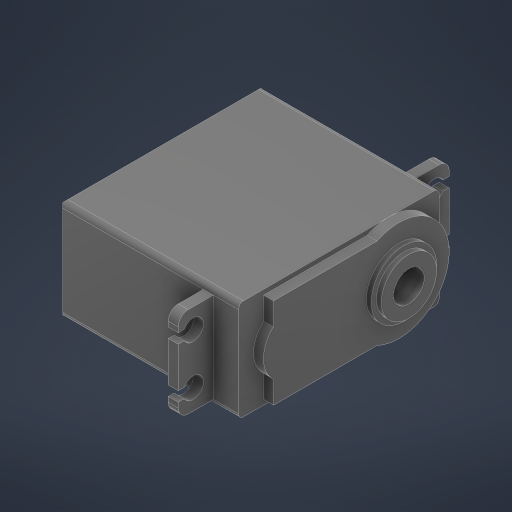
# Autodesk Inventor part: Servo
Saved by Autodesk Inventor 2023.2 (Build 272271000, 271)
## iProperties
Created: 2023-04-06
Part Number: Servo
Material: ABS-Kunststoff
Document SubType Name: Modeling
Designer: tadeus
Density: 1.06 g/cm^3
Appearance: Glatt - Weiß
Author: tadeus
Autodesk Inventor part; units mm, degrees
ref_plane "YZ Plane" through (0, 0, 0) normal (1, 0, 0) x (0, 1, 0)
ref_plane "XZ Plane" through (0, 0, 0) normal (0, 1, 0) x (-1, 0, 0)
ref_plane "XY Plane" through (0, 0, 0) normal (0, 0, 1) x (1, 0, 0)
sketch "Skizze1" plane through (0, 0, 0) normal (0, 1, 0) x (-1, 0, 0)
  line L0 (18.5, -20) -> (-18.5, -20)
  line L1 (-18.5, -20) -> (-18.5, 20)
  line L2 (-18.5, 20) -> (18.5, 20)
  line L3 (18.5, 20) -> (18.5, -20)
  line L4 (18.5, -20) -> (-18.5, 20) construction
  line L5 (-18.5, -20) -> (18.5, 20) construction
  point P0 (0, 0)
  dimension "d0" = 37
  dimension "d1" = 40
  constraints: 12 end point, 2 midpoint, 2 parallel, 1 horizontal, 1 perpendicular
  measures "d0" distance of L1.end L2.end
  measures "d1" distance of L0.end L1.end
extrude "Extrusion1" add sketch "Skizze1" along normal blind 20
sketch "Skizze2" plane through (0, 0, 0) normal (0, 0, 1) x (1, 0, 0)
  line L0 (-14.5, 13.5) -> (-10.5, 13.5)
  line L1 (-10.5, 13.5) -> (-10.5, 6.5)
  line L2 (-10.5, 6.5) -> (-14.5, 6.5)
  line L3 (-14.5, 6.5) -> (-14.5, 13.5)
  line L4 (-14.5, 13.5) -> (-10.5, 6.5) construction
  line L5 (-10.5, 13.5) -> (-14.5, 6.5) construction
  line L6 (-18.5, 20) -> (18.5, 20) projected
  line L7 (-18.5, 0) -> (-18.5, 20) projected
  line L8 (11.5, 19) -> (13.5, 19)
  line L9 (13.5, 19) -> (13.5, 1)
  line L10 (13.5, 1) -> (11.5, 1)
  line L11 (11.5, 1) -> (11.5, 19)
  line L12 (11.5, 19) -> (13.5, 1) construction
  line L13 (13.5, 19) -> (11.5, 1) construction
  line L14 (18.5, 0) -> (18.5, 20) projected
  point P0 (0, 0)
  point P1 (-12.5, 10)
  point P2 (12.5, 10)
  point P3 (18.5, 10)
  dimension "d4" = 4
  dimension "d5" = 7
  dimension "d6" = 10
  dimension "d7" = 6
  dimension "d10" = 2
  dimension "d11" = 18
  dimension "d12" = 6
  constraints: 24 end point, 5 midpoint, 4 parallel, 2 horizontal, 2 perpendicular
  measures "d4" distance of L1.end L2.end
  measures "d5" distance of L0.end L1.end
  measures "d6" distance from line of L6 point (-12.5, 10)
  measures "d7" distance from line of L7 point (-12.5, 10)
  measures "d10" distance of L9.end L10.end
  measures "d11" distance of L8.end L9.end
  measures "d12" distance of point (18.5, 10) point (12.5, 10)
extrude "Extrusion2" add sketch "Skizze2" against normal blind 5 from surface at -20 contours L0 L1 L2 L3
extrude "Extrusion3" add sketch "Skizze2" along normal mid plane 54 contours L8 L9 L10 L11
sketch "Skizze3" plane through (0, 0, 0) normal (1, 0, 0) x (0, 1, 0)
  arc A0 (15, 26.05) -> (14, 25.7896) centre (15, 24) ccw construction
  arc A1 (4, 25.7896) -> (6, 25.7896) centre (5, 24) ccw
  line L0 (1, 27) -> (19, 27) construction
  line L1 (15, 24) -> (5, 24) construction
  line L2 (19, 20) -> (19, 27) projected
  line L3 (-8.9518, 0) -> (31.8081, 0) construction
  line L4 (15, 24) -> (15, 27) construction
  line L5 (16, 25.1) -> (14, 25.1) construction
  line L6 (14, 25.1) -> (14, 25.7896)
  line L7 (14, 27) -> (16, 27)
  line L8 (16, 27) -> (16, 25.7896)
  line L9 (16, 25.1) -> (14, 27) construction
  line L10 (14, 25.1) -> (16, 27) construction
  line L11 (5, 24) -> (5, 27) construction
  line L12 (6, 25.1) -> (4, 25.1) construction
  line L13 (4, 25.1) -> (4, 25.7896) construction
  line L14 (4, 27) -> (6, 27)
  line L15 (6, 27) -> (6, 25.7896)
  line L16 (6, 25.1) -> (4, 27) construction
  line L17 (4, 25.1) -> (6, 27) construction
  line L18 (16, 25.7896) -> (16, 25.1) construction
  line L19 (14, 25.7896) -> (14, 27)
  arc A2 (16, 25.7896) -> (15, 26.05) centre (15, 24) ccw construction
  arc A3 (14, 25.7896) -> (16, 25.7896) centre (15, 24) ccw
  line L20 (6, 25.7896) -> (6, 25.1) construction
  line L21 (4, 25.7896) -> (4, 27)
  arc A4 (5, 26.05) -> (4, 25.7896) centre (5, 24) ccw construction
  arc A5 (6, 25.7896) -> (5, 26.05) centre (5, 24) ccw construction
  arc A6 (6, -25.7896) -> (4, -25.7896) centre (5, -24) ccw
  line L22 (14, -27) -> (16, -27)
  line L23 (16, -27) -> (16, -25.7896)
  line L24 (4, -27) -> (6, -27)
  line L25 (6, -27) -> (6, -25.7896)
  line L26 (14, -25.7896) -> (14, -27)
  arc A7 (16, -25.7896) -> (14, -25.7896) centre (15, -24) ccw
  line L27 (4, -25.7896) -> (4, -27)
  arc A8 (1, -5.6411) -> (19, -5.6411) centre (10, -10) ccw
  line L28 (20, 20) -> (20, -20) projected
  line L29 (0, -20) -> (20, -20) projected
  line L30 (19, -15) -> (1, -15) construction
  line L31 (1, -15) -> (1, -5.6411) construction
  line L32 (1, 15) -> (5.5, 15)
  line L33 (19, 15) -> (19, -5.6411)
  line L34 (19, -15) -> (1, 15) construction
  line L35 (1, -15) -> (19, 15) construction
  line L36 (0, 20) -> (20, 20) projected
  line L37 (19, -5.6411) -> (19, -15) construction
  line L38 (1, -5.6411) -> (1, 15)
  arc A9 (10, 0) -> (1, -5.6411) centre (10, -10) ccw construction
  arc A10 (19, -5.6411) -> (10, 0) centre (10, -10) ccw construction
  arc A11 (14.5, 15) -> (5.5, 15) centre (10, 10.9375) ccw
  line L39 (5.5, 15) -> (14.5, 15) construction
  line L40 (14.5, 15) -> (19, 15)
  point P0 (0, 0)
  point P1 (10, 15)
  point P2 (10, 17)
  dimension "d15" = 4.1
  dimension "d16" = 4.1
  dimension "d17" = 10
  dimension "d21" = 24
  dimension "d22" = 4
  dimension "d23" = 2
  dimension "d24" = 2
  dimension "d27" = 20
  dimension "d28" = 10
  dimension "d29" = 10
  dimension "d30" = 18
  dimension "d31" = 5
  dimension "d32" = 9
  dimension "d35" = 9
  dimension "d36" = 4.5
  dimension "d38" = 2
  constraints: 72 end point, 25 point on circle, 17 parallel, 12 centre point, 10 midpoint, 10 symmetric about line, 9 point on line, 8 perpendicular, 6 horizontal, 2 other
  measures "d15" diameter of A0
  measures "d16" diameter of A1
  measures "d17" distance of L1.end L1.start
  measures "d21" vertical distance of L1.end point (0, 0)
  measures "d22" distance from line of L2 L1.start
  measures "d23" distance of L7.start L7.end
  measures "d24" distance of L14.start L14.end
  measures "d27" diameter of A8
  measures "d28" distance from line of L28 A8.centre
  measures "d29" distance from line of L29 A8.centre
  measures "d30" distance of L32.start L33.start
  measures "d31" distance between parallel lines of L36 L32
  measures "d32" distance of L33.start point (10, 15)
  measures "d35" distance of L32.end L39.end
  measures "d36" distance of point (10, 15) L39.end
  measures "d38" distance from line of L32 point (10, 17)
extrude "Extrusion4" cut sketch "Skizze3" along normal through all contours L21 L14 L15 A1 | L7 L8 A3 L19 | L25 L24 L27 A6 | L26 A7 L23 L22
extrude "Extrusion5" add sketch "Skizze3" along normal blind 2 from surface at 18.5 contours L38 L32 A11 L40 L33 A8
sketch "Skizze4" plane through (20.5, 10, -10) normal (1, 0, 0) x (0, 0, -1)
  circle A0 centre (0, 0) radius 6.5
  circle A1 centre (0, 0) radius 5.5
  arc A2 (-4.3589, -9) -> (-4.3589, 9) centre (0, 0) ccw construction
  line L0 (0, 10) -> (10, 10) construction
  line L1 (0, 2.75) -> (0, 3) construction
  line L2 (-0.3447, 2.7283) -> (-0.376, 2.9763) construction
  line L3 (-0.6839, 2.6636) -> (-0.7461, 2.9057) construction
  line L4 (-1.0123, 2.5569) -> (-1.1044, 2.7893) construction
  line L5 (-1.3248, 2.4098) -> (-1.4453, 2.6289) construction
  line L6 (-1.6164, 2.2248) -> (-1.7634, 2.4271) construction
  line L7 (-1.8825, 2.0047) -> (-2.0536, 2.1869) construction
  line L8 (-2.1189, 1.7529) -> (-2.3115, 1.9123) construction
  line L9 (-2.3219, 1.4735) -> (-2.533, 1.6075) construction
  line L10 (-2.4883, 1.1709) -> (-2.7145, 1.2773) construction
  line L11 (-2.6154, 0.8498) -> (-2.8532, 0.9271) construction
  line L12 (-2.7013, 0.5153) -> (-2.9469, 0.5621) construction
  line L13 (-2.7446, 0.1727) -> (-2.9941, 0.1884) construction
  line L14 (-2.7446, -0.1727) -> (-2.9941, -0.1884) construction
  line L15 (-2.7013, -0.5153) -> (-2.9469, -0.5621) construction
  line L16 (-2.6154, -0.8498) -> (-2.8532, -0.9271) construction
  line L17 (-2.4883, -1.1709) -> (-2.7145, -1.2773) construction
  line L18 (-2.3219, -1.4735) -> (-2.533, -1.6075) construction
  line L19 (-2.1189, -1.7529) -> (-2.3115, -1.9123) construction
  line L20 (-1.8825, -2.0047) -> (-2.0536, -2.1869) construction
  line L21 (-1.6164, -2.2248) -> (-1.7634, -2.4271) construction
  line L22 (-1.3248, -2.4098) -> (-1.4453, -2.6289) construction
  line L23 (-1.0123, -2.5569) -> (-1.1044, -2.7893) construction
  line L24 (-0.6839, -2.6636) -> (-0.7461, -2.9057) construction
  line L25 (-0.3447, -2.7283) -> (-0.376, -2.9763) construction
  line L26 (0, -2.75) -> (0, -3) construction
  line L27 (0.3447, -2.7283) -> (0.376, -2.9763) construction
  line L28 (0.6839, -2.6636) -> (0.7461, -2.9057) construction
  line L29 (1.0123, -2.5569) -> (1.1044, -2.7893) construction
  line L30 (1.3248, -2.4098) -> (1.4453, -2.6289) construction
  line L31 (1.6164, -2.2248) -> (1.7634, -2.4271) construction
  line L32 (1.8825, -2.0047) -> (2.0536, -2.1869) construction
  line L33 (2.1189, -1.7529) -> (2.3115, -1.9123) construction
  line L34 (2.3219, -1.4735) -> (2.533, -1.6075) construction
  line L35 (2.4883, -1.1709) -> (2.7145, -1.2773) construction
  line L36 (2.6154, -0.8498) -> (2.8532, -0.9271) construction
  line L37 (2.7013, -0.5153) -> (2.9469, -0.5621) construction
  line L38 (2.7446, -0.1727) -> (2.9941, -0.1884) construction
  line L39 (2.7446, 0.1727) -> (2.9941, 0.1884) construction
  line L40 (2.7013, 0.5153) -> (2.9469, 0.5621) construction
  line L41 (2.6154, 0.8498) -> (2.8532, 0.9271) construction
  line L42 (2.4883, 1.1709) -> (2.7145, 1.2773) construction
  line L43 (2.3219, 1.4735) -> (2.533, 1.6075) construction
  line L44 (2.1189, 1.7529) -> (2.3115, 1.9123) construction
  line L45 (1.8825, 2.0047) -> (2.0536, 2.1869) construction
  line L46 (1.6164, 2.2248) -> (1.7634, 2.4271) construction
  line L47 (1.3248, 2.4098) -> (1.4453, 2.6289) construction
  line L48 (1.0123, 2.5569) -> (1.1044, 2.7893) construction
  line L49 (0.6839, 2.6636) -> (0.7461, 2.9057) construction
  line L50 (0.3447, 2.7283) -> (0.376, 2.9763) construction
  spline S0 degree 4 poles (0, 3) (0.1244, 3) (0.1756, 2.8504) (0.2331, 2.7424) (0.3447, 2.7283) knots 0 0 0 0 0 1 1 1 1 1
  line L51 (0.3012, 2.7338) -> (0.3881, 2.7228) construction
  arc A3 (0.3111, 2.7361) -> (0.3791, 2.7275) centre (0.3658, 2.8957) ccw construction
  line L52 (-0.0449, 3) -> (0.0449, 3) construction
  arc A4 (0.0348, 2.9956) -> (-0.0348, 2.9956) centre (0, 2.862) ccw construction
  spline S1 degree 4 poles (0, 3) (-0.1244, 3) (-0.1756, 2.8504) (-0.2331, 2.7424) (-0.3447, 2.7283) knots 0 0 0 0 0 1 1 1 1 1
  line L53 (-0.3012, 2.7338) -> (-0.3881, 2.7228) construction
  arc A5 (-0.3791, 2.7275) -> (-0.3111, 2.7361) centre (-0.3658, 2.8957) ccw construction
  line L54 (0.0449, 3) -> (-0.0449, 3) construction
  arc A6 (0.0348, 2.9956) -> (-0.0348, 2.9956) centre (0, 2.862) ccw construction
  spline S2 degree 4 poles (-0.7461, 2.9057) (-0.6256, 2.9367) (-0.5388, 2.8045) (-0.4562, 2.7142) (-0.3447, 2.7283) knots 0 0 0 0 0 1 1 1 1 1
  line L55 (-0.3881, 2.7228) -> (-0.3012, 2.7338) construction
  line L56 (-0.7895, 2.8946) -> (-0.7026, 2.9169) construction
  arc A7 (-0.3791, 2.7275) -> (-0.3111, 2.7361) centre (-0.3658, 2.8957) ccw construction
  arc A8 (-0.7113, 2.9101) -> (-0.7786, 2.8928) centre (-0.7118, 2.7721) ccw construction
  spline S3 degree 4 poles (-0.7461, 2.9057) (-0.8666, 2.8748) (-0.879, 2.7172) (-0.9078, 2.5983) (-1.0123, 2.5569) knots 0 0 0 0 0 1 1 1 1 1
  line L57 (-0.9716, 2.573) -> (-1.0531, 2.5408) construction
  line L58 (-0.7026, 2.9169) -> (-0.7895, 2.8946) construction
  arc A9 (-1.0455, 2.5475) -> (-0.9817, 2.5728) centre (-1.0745, 2.7138) ccw construction
  arc A10 (-0.7113, 2.9101) -> (-0.7786, 2.8928) centre (-0.7118, 2.7721) ccw construction
  spline S4 degree 4 poles (-1.4453, 2.6289) (-1.3362, 2.6889) (-1.2193, 2.5824) (-1.1169, 2.5155) (-1.0123, 2.5569) knots 0 0 0 0 0 1 1 1 1 1
  line L59 (-1.0531, 2.5408) -> (-0.9716, 2.573) construction
  line L60 (-1.4846, 2.6073) -> (-1.4059, 2.6505) construction
  arc A11 (-1.0455, 2.5475) -> (-0.9817, 2.5728) centre (-1.0745, 2.7138) ccw construction
  arc A12 (-1.4127, 2.6418) -> (-1.4736, 2.6083) centre (-1.3788, 2.508) ccw construction
  spline S5 degree 4 poles (-1.4453, 2.6289) (-1.5543, 2.569) (-1.5271, 2.4132) (-1.5254, 2.2909) (-1.6164, 2.2248) knots 0 0 0 0 0 1 1 1 1 1
  line L61 (-1.581, 2.2505) -> (-1.6518, 2.1991) construction
  line L62 (-1.4059, 2.6505) -> (-1.4846, 2.6073) construction
  arc A13 (-1.6462, 2.2075) -> (-1.5907, 2.2478) centre (-1.7156, 2.3613) ccw construction
  arc A14 (-1.4127, 2.6418) -> (-1.4736, 2.6083) centre (-1.3788, 2.508) ccw construction
  spline S6 degree 4 poles (-2.0536, 2.1869) (-1.9629, 2.2721) (-1.8232, 2.1981) (-1.7074, 2.1587) (-1.6164, 2.2248) knots 0 0 0 0 0 1 1 1 1 1
  line L63 (-1.6518, 2.1991) -> (-1.581, 2.2505) construction
  line L64 (-2.0864, 2.1562) -> (-2.0209, 2.2176) construction
  arc A15 (-1.6462, 2.2075) -> (-1.5907, 2.2478) centre (-1.7156, 2.3613) ccw construction
  arc A16 (-2.0253, 2.2075) -> (-2.0759, 2.1599) centre (-1.9592, 2.0863) ccw construction
  spline S7 degree 4 poles (-2.0536, 2.1869) (-2.1443, 2.1017) (-2.0792, 1.9576) (-2.0472, 1.8396) (-2.1189, 1.7529) knots 0 0 0 0 0 1 1 1 1 1
  line L65 (-2.091, 1.7867) -> (-2.1468, 1.7192) construction
  line L66 (-2.0209, 2.2176) -> (-2.0864, 2.1562) construction
  arc A17 (-2.1435, 1.7287) -> (-2.0998, 1.7816) centre (-2.2489, 1.8605) ccw construction
  arc A18 (-2.0253, 2.2075) -> (-2.0759, 2.1599) centre (-1.9592, 2.0863) ccw construction
  spline S8 degree 4 poles (-2.533, 1.6075) (-2.4663, 1.7125) (-2.3126, 1.6756) (-2.1906, 1.6663) (-2.1189, 1.7529) knots 0 0 0 0 0 1 1 1 1 1
  line L67 (-2.1468, 1.7192) -> (-2.091, 1.7867) construction
  line L68 (-2.557, 1.5696) -> (-2.5089, 1.6454) construction
  arc A19 (-2.1435, 1.7287) -> (-2.0998, 1.7816) centre (-2.2489, 1.8605) ccw construction
  arc A20 (-2.5106, 1.6344) -> (-2.5478, 1.5758) centre (-2.4165, 1.5335) ccw construction
  spline S9 degree 4 poles (-2.533, 1.6075) (-2.5997, 1.5024) (-2.5008, 1.3791) (-2.4404, 1.2727) (-2.4883, 1.1709) knots 0 0 0 0 0 1 1 1 1 1
  line L69 (-2.4696, 1.2105) -> (-2.5069, 1.1313) construction
  line L70 (-2.5089, 1.6454) -> (-2.557, 1.5696) construction
  arc A21 (-2.5061, 1.1414) -> (-2.4769, 1.2034) centre (-2.641, 1.2427) ccw construction
  arc A22 (-2.5106, 1.6344) -> (-2.5478, 1.5758) centre (-2.4165, 1.5335) ccw construction
  spline S10 degree 4 poles (-2.8532, 0.9271) (-2.8147, 1.0454) (-2.6566, 1.0478) (-2.5362, 1.0691) (-2.4883, 1.1709) knots 0 0 0 0 0 1 1 1 1 1
  line L71 (-2.5069, 1.1313) -> (-2.4696, 1.2105) construction
  line L72 (-2.867, 0.8844) -> (-2.8393, 0.9697) construction
  arc A23 (-2.5061, 1.1414) -> (-2.4769, 1.2034) centre (-2.641, 1.2427) ccw construction
  arc A24 (-2.8382, 0.9587) -> (-2.8597, 0.8926) centre (-2.7219, 0.8844) ccw construction
  spline S11 degree 4 poles (-2.8532, 0.9271) (-2.8916, 0.8087) (-2.7652, 0.7138) (-2.6802, 0.6258) (-2.7013, 0.5153) knots 0 0 0 0 0 1 1 1 1 1
  line L73 (-2.6931, 0.5583) -> (-2.7095, 0.4723) construction
  line L74 (-2.8393, 0.9697) -> (-2.867, 0.8844) construction
  arc A25 (-2.7112, 0.4823) -> (-2.6983, 0.5497) centre (-2.867, 0.5469) ccw construction
  arc A26 (-2.8382, 0.9587) -> (-2.8597, 0.8926) centre (-2.7219, 0.8844) ccw construction
  spline S12 degree 4 poles (-2.9941, 0.1884) (-2.9863, 0.3125) (-2.8338, 0.3542) (-2.7224, 0.4048) (-2.7013, 0.5153) knots 0 0 0 0 0 1 1 1 1 1
  line L75 (-2.7095, 0.4723) -> (-2.6931, 0.5583) construction
  line L76 (-2.9969, 0.1436) -> (-2.9913, 0.2332) construction
  arc A27 (-2.7112, 0.4823) -> (-2.6983, 0.5497) centre (-2.867, 0.5469) ccw construction
  arc A28 (-2.9875, 0.2228) -> (-2.9918, 0.1534) centre (-2.8564, 0.1797) ccw construction
  spline S13 degree 4 poles (-2.9941, 0.1884) (-3.0019, 0.0642) (-2.8558, 0.0037) (-2.7516, -0.0604) (-2.7446, -0.1727) knots 0 0 0 0 0 1 1 1 1 1
  line L77 (-2.7473, -0.129) -> (-2.7418, -0.2164) construction
  line L78 (-2.9913, 0.2332) -> (-2.9969, 0.1436) construction
  arc A29 (-2.7459, -0.2071) -> (-2.7502, -0.1387) centre (-2.913, -0.1833) ccw construction
  arc A30 (-2.9875, 0.2228) -> (-2.9918, 0.1534) centre (-2.8564, 0.1797) ccw construction
  spline S14 degree 4 poles (-2.9469, -0.5621) (-2.9702, -0.4399) (-2.8328, -0.3616) (-2.7375, -0.2849) (-2.7446, -0.1727) knots 0 0 0 0 0 1 1 1 1 1
  line L79 (-2.7418, -0.2164) -> (-2.7473, -0.129) construction
  line L80 (-2.9385, -0.6062) -> (-2.9553, -0.518) construction
  arc A31 (-2.7459, -0.2071) -> (-2.7502, -0.1387) centre (-2.913, -0.1833) ccw construction
  arc A32 (-2.949, -0.5272) -> (-2.936, -0.5954) centre (-2.8113, -0.5363) ccw construction
  spline S15 degree 4 poles (-2.9469, -0.5621) (-2.9235, -0.6844) (-2.767, -0.7066) (-2.6502, -0.7428) (-2.6154, -0.8498) knots 0 0 0 0 0 1 1 1 1 1
  line L81 (-2.6289, -0.8081) -> (-2.6019, -0.8914) construction
  line L82 (-2.9553, -0.518) -> (-2.9385, -0.6062) construction
  arc A33 (-2.6082, -0.8835) -> (-2.6294, -0.8183) centre (-2.7759, -0.9019) ccw construction
  arc A34 (-2.949, -0.5272) -> (-2.936, -0.5954) centre (-2.8113, -0.5363) ccw construction
  spline S16 degree 4 poles (-2.7145, -1.2773) (-2.7675, -1.1648) (-2.6539, -1.0548) (-2.5807, -0.9568) (-2.6154, -0.8498) knots 0 0 0 0 0 1 1 1 1 1
  line L83 (-2.6019, -0.8914) -> (-2.6289, -0.8081) construction
  line L84 (-2.6954, -1.318) -> (-2.7336, -1.2367) construction
  arc A35 (-2.6082, -0.8835) -> (-2.6294, -0.8183) centre (-2.7759, -0.9019) ccw construction
  arc A36 (-2.7253, -1.244) -> (-2.6957, -1.3069) centre (-2.5896, -1.2186) ccw construction
  spline S17 degree 4 poles (-2.7145, -1.2773) (-2.6615, -1.3899) (-2.5044, -1.3725) (-2.3822, -1.3786) (-2.3219, -1.4735) knots 0 0 0 0 0 1 1 1 1 1
  line L85 (-2.3454, -1.4365) -> (-2.2984, -1.5105) construction
  line L86 (-2.7336, -1.2367) -> (-2.6954, -1.318) construction
  arc A37 (-2.3065, -1.5044) -> (-2.3433, -1.4464) centre (-2.4644, -1.5639) ccw construction
  arc A38 (-2.7253, -1.244) -> (-2.6957, -1.3069) centre (-2.5896, -1.2186) ccw construction
  spline S18 degree 4 poles (-2.3115, -1.9123) (-2.3908, -1.8164) (-2.3082, -1.6816) (-2.2616, -1.5685) (-2.3219, -1.4735) knots 0 0 0 0 0 1 1 1 1 1
  line L87 (-2.2984, -1.5105) -> (-2.3454, -1.4365) construction
  line L88 (-2.2829, -1.9469) -> (-2.3402, -1.8777) construction
  arc A39 (-2.3065, -1.5044) -> (-2.3433, -1.4464) centre (-2.4644, -1.5639) ccw construction
  arc A40 (-2.3303, -1.8827) -> (-2.286, -1.9362) centre (-2.2052, -1.8243) ccw construction
  spline S19 degree 4 poles (-2.3115, -1.9123) (-2.2322, -2.0081) (-2.0843, -1.9522) (-1.9645, -1.9277) (-1.8825, -2.0047) knots 0 0 0 0 0 1 1 1 1 1
  line L89 (-1.9144, -1.9747) -> (-1.8506, -2.0346) construction
  line L90 (-2.3402, -1.8777) -> (-2.2829, -1.9469) construction
  arc A41 (-1.8599, -2.0307) -> (-1.9099, -1.9838) centre (-1.998, -2.1277) ccw construction
  arc A42 (-2.3303, -1.8827) -> (-2.286, -1.9362) centre (-2.2052, -1.8243) ccw construction
  spline S20 degree 4 poles (-1.7634, -2.4271) (-1.864, -2.3539) (-1.8175, -2.2028) (-1.8005, -2.0817) (-1.8825, -2.0047) knots 0 0 0 0 0 1 1 1 1 1
  line L91 (-1.8506, -2.0346) -> (-1.9144, -1.9747) construction
  line L92 (-1.727, -2.4534) -> (-1.7997, -2.4007) construction
  arc A43 (-1.8599, -2.0307) -> (-1.9099, -1.9838) centre (-1.998, -2.1277) ccw construction
  arc A44 (-1.7889, -2.403) -> (-1.7326, -2.4439) centre (-1.6823, -2.3154) ccw construction
  spline S21 degree 4 poles (-1.7634, -2.4271) (-1.6627, -2.5002) (-1.5334, -2.4092) (-1.4234, -2.3557) (-1.3248, -2.4098) knots 0 0 0 0 0 1 1 1 1 1
  line L93 (-1.3632, -2.3887) -> (-1.2864, -2.4309) construction
  line L94 (-1.7997, -2.4007) -> (-1.727, -2.4534) construction
  arc A45 (-1.2965, -2.4295) -> (-1.3566, -2.3964) centre (-1.4061, -2.5577) ccw construction
  arc A46 (-1.7889, -2.403) -> (-1.7326, -2.4439) centre (-1.6823, -2.3154) ccw construction
  spline S22 degree 4 poles (-1.1044, -2.7893) (-1.2201, -2.7435) (-1.2126, -2.5856) (-1.2263, -2.464) (-1.3248, -2.4098) knots 0 0 0 0 0 1 1 1 1 1
  line L95 (-1.2864, -2.4309) -> (-1.3632, -2.3887) construction
  line L96 (-1.0626, -2.8059) -> (-1.1461, -2.7728) construction
  arc A47 (-1.2965, -2.4295) -> (-1.3566, -2.3964) centre (-1.4061, -2.5577) ccw construction
  arc A48 (-1.135, -2.7724) -> (-1.0704, -2.798) centre (-1.0536, -2.661) ccw construction
  spline S23 degree 4 poles (-1.1044, -2.7893) (-0.9887, -2.8351) (-0.886, -2.7149) (-0.7928, -2.6356) (-0.6839, -2.6636) knots 0 0 0 0 0 1 1 1 1 1
  line L97 (-0.7263, -2.6527) -> (-0.6415, -2.6745) construction
  line L98 (-1.1461, -2.7728) -> (-1.0626, -2.8059) construction
  arc A49 (-0.6515, -2.6755) -> (-0.718, -2.6585) centre (-0.7259, -2.827) ccw construction
  arc A50 (-1.135, -2.7724) -> (-1.0704, -2.798) centre (-1.0536, -2.661) ccw construction
  spline S24 degree 4 poles (-0.376, -2.9763) (-0.4994, -2.9607) (-0.5315, -2.8059) (-0.575, -2.6916) (-0.6839, -2.6636) knots 0 0 0 0 0 1 1 1 1 1
  line L99 (-0.6415, -2.6745) -> (-0.7263, -2.6527) construction
  line L100 (-0.3315, -2.982) -> (-0.4205, -2.9707) construction
  arc A51 (-0.6515, -2.6755) -> (-0.718, -2.6585) centre (-0.7259, -2.827) ccw construction
  arc A52 (-0.4099, -2.9676) -> (-0.341, -2.9763) centre (-0.3587, -2.8395) ccw construction
  spline S25 degree 4 poles (-0.376, -2.9763) (-0.2526, -2.9919) (-0.183, -2.8499) (-0.1125, -2.75) (0, -2.75) knots 0 0 0 0 0 1 1 1 1 1
  line L101 (-0.0438, -2.75) -> (0.0438, -2.75) construction
  line L102 (-0.4205, -2.9707) -> (-0.3315, -2.982) construction
  arc A53 (0.0343, -2.7535) -> (-0.0343, -2.7535) centre (0, -2.9187) ccw construction
  arc A54 (-0.4099, -2.9676) -> (-0.341, -2.9763) centre (-0.3587, -2.8395) ccw construction
  spline S26 degree 4 poles (0.376, -2.9763) (0.2526, -2.9919) (0.183, -2.8499) (0.1125, -2.75) (0, -2.75) knots 0 0 0 0 0 1 1 1 1 1
  line L103 (0.0438, -2.75) -> (-0.0438, -2.75) construction
  line L104 (0.4205, -2.9707) -> (0.3315, -2.982) construction
  arc A55 (0.0343, -2.7535) -> (-0.0343, -2.7535) centre (0, -2.9187) ccw construction
  arc A56 (0.341, -2.9763) -> (0.4099, -2.9676) centre (0.3587, -2.8395) ccw construction
  spline S27 degree 4 poles (0.376, -2.9763) (0.4994, -2.9607) (0.5315, -2.8059) (0.575, -2.6916) (0.6839, -2.6636) knots 0 0 0 0 0 1 1 1 1 1
  line L105 (0.6415, -2.6745) -> (0.7263, -2.6527) construction
  line L106 (0.3315, -2.982) -> (0.4205, -2.9707) construction
  arc A57 (0.718, -2.6585) -> (0.6515, -2.6755) centre (0.7259, -2.827) ccw construction
  arc A58 (0.341, -2.9763) -> (0.4099, -2.9676) centre (0.3587, -2.8395) ccw construction
  spline S28 degree 4 poles (1.1044, -2.7893) (0.9887, -2.8351) (0.886, -2.7149) (0.7928, -2.6356) (0.6839, -2.6636) knots 0 0 0 0 0 1 1 1 1 1
  line L107 (0.7263, -2.6527) -> (0.6415, -2.6745) construction
  line L108 (1.1461, -2.7728) -> (1.0626, -2.8059) construction
  arc A59 (0.718, -2.6585) -> (0.6515, -2.6755) centre (0.7259, -2.827) ccw construction
  arc A60 (1.0704, -2.798) -> (1.135, -2.7724) centre (1.0536, -2.661) ccw construction
  spline S29 degree 4 poles (1.1044, -2.7893) (1.2201, -2.7435) (1.2126, -2.5856) (1.2263, -2.464) (1.3248, -2.4098) knots 0 0 0 0 0 1 1 1 1 1
  line L109 (1.2864, -2.4309) -> (1.3632, -2.3887) construction
  line L110 (1.0626, -2.8059) -> (1.1461, -2.7728) construction
  arc A61 (1.3566, -2.3964) -> (1.2965, -2.4295) centre (1.4061, -2.5577) ccw construction
  arc A62 (1.0704, -2.798) -> (1.135, -2.7724) centre (1.0536, -2.661) ccw construction
  spline S30 degree 4 poles (1.7634, -2.4271) (1.6627, -2.5002) (1.5334, -2.4092) (1.4234, -2.3557) (1.3248, -2.4098) knots 0 0 0 0 0 1 1 1 1 1
  line L111 (1.3632, -2.3887) -> (1.2864, -2.4309) construction
  line L112 (1.7997, -2.4007) -> (1.727, -2.4534) construction
  arc A63 (1.3566, -2.3964) -> (1.2965, -2.4295) centre (1.4061, -2.5577) ccw construction
  arc A64 (1.7326, -2.4439) -> (1.7889, -2.403) centre (1.6823, -2.3154) ccw construction
  spline S31 degree 4 poles (1.7634, -2.4271) (1.864, -2.3539) (1.8175, -2.2028) (1.8005, -2.0817) (1.8825, -2.0047) knots 0 0 0 0 0 1 1 1 1 1
  line L113 (1.8506, -2.0346) -> (1.9144, -1.9747) construction
  line L114 (1.727, -2.4534) -> (1.7997, -2.4007) construction
  arc A65 (1.9099, -1.9838) -> (1.8599, -2.0307) centre (1.998, -2.1277) ccw construction
  arc A66 (1.7326, -2.4439) -> (1.7889, -2.403) centre (1.6823, -2.3154) ccw construction
  spline S32 degree 4 poles (2.3115, -1.9123) (2.2322, -2.0081) (2.0843, -1.9522) (1.9645, -1.9277) (1.8825, -2.0047) knots 0 0 0 0 0 1 1 1 1 1
  line L115 (1.9144, -1.9747) -> (1.8506, -2.0346) construction
  line L116 (2.3402, -1.8777) -> (2.2829, -1.9469) construction
  arc A67 (1.9099, -1.9838) -> (1.8599, -2.0307) centre (1.998, -2.1277) ccw construction
  arc A68 (2.286, -1.9362) -> (2.3303, -1.8827) centre (2.2052, -1.8243) ccw construction
  spline S33 degree 4 poles (2.3115, -1.9123) (2.3908, -1.8164) (2.3082, -1.6816) (2.2616, -1.5685) (2.3219, -1.4735) knots 0 0 0 0 0 1 1 1 1 1
  line L117 (2.2984, -1.5105) -> (2.3454, -1.4365) construction
  line L118 (2.2829, -1.9469) -> (2.3402, -1.8777) construction
  arc A69 (2.3433, -1.4464) -> (2.3065, -1.5044) centre (2.4644, -1.5639) ccw construction
  arc A70 (2.286, -1.9362) -> (2.3303, -1.8827) centre (2.2052, -1.8243) ccw construction
  spline S34 degree 4 poles (2.7145, -1.2773) (2.6615, -1.3899) (2.5044, -1.3725) (2.3822, -1.3786) (2.3219, -1.4735) knots 0 0 0 0 0 1 1 1 1 1
  line L119 (2.3454, -1.4365) -> (2.2984, -1.5105) construction
  line L120 (2.7336, -1.2367) -> (2.6954, -1.318) construction
  arc A71 (2.3433, -1.4464) -> (2.3065, -1.5044) centre (2.4644, -1.5639) ccw construction
  arc A72 (2.6957, -1.3069) -> (2.7253, -1.244) centre (2.5896, -1.2186) ccw construction
  spline S35 degree 4 poles (2.7145, -1.2773) (2.7675, -1.1648) (2.6539, -1.0548) (2.5807, -0.9568) (2.6154, -0.8498) knots 0 0 0 0 0 1 1 1 1 1
  line L121 (2.6019, -0.8914) -> (2.6289, -0.8081) construction
  line L122 (2.6954, -1.318) -> (2.7336, -1.2367) construction
  arc A73 (2.6294, -0.8183) -> (2.6082, -0.8835) centre (2.7759, -0.9019) ccw construction
  arc A74 (2.6957, -1.3069) -> (2.7253, -1.244) centre (2.5896, -1.2186) ccw construction
  spline S36 degree 4 poles (2.9469, -0.5621) (2.9235, -0.6844) (2.767, -0.7066) (2.6502, -0.7428) (2.6154, -0.8498) knots 0 0 0 0 0 1 1 1 1 1
  line L123 (2.6289, -0.8081) -> (2.6019, -0.8914) construction
  line L124 (2.9553, -0.518) -> (2.9385, -0.6062) construction
  arc A75 (2.6294, -0.8183) -> (2.6082, -0.8835) centre (2.7759, -0.9019) ccw construction
  arc A76 (2.936, -0.5954) -> (2.949, -0.5272) centre (2.8113, -0.5363) ccw construction
  spline S37 degree 4 poles (2.9469, -0.5621) (2.9702, -0.4399) (2.8328, -0.3616) (2.7375, -0.2849) (2.7446, -0.1727) knots 0 0 0 0 0 1 1 1 1 1
  line L125 (2.7418, -0.2164) -> (2.7473, -0.129) construction
  line L126 (2.9385, -0.6062) -> (2.9553, -0.518) construction
  arc A77 (2.7502, -0.1387) -> (2.7459, -0.2071) centre (2.913, -0.1833) ccw construction
  arc A78 (2.936, -0.5954) -> (2.949, -0.5272) centre (2.8113, -0.5363) ccw construction
  spline S38 degree 4 poles (2.9941, 0.1884) (3.0019, 0.0642) (2.8558, 0.0037) (2.7516, -0.0604) (2.7446, -0.1727) knots 0 0 0 0 0 1 1 1 1 1
  line L127 (2.7473, -0.129) -> (2.7418, -0.2164) construction
  line L128 (2.9913, 0.2332) -> (2.9969, 0.1436) construction
  arc A79 (2.7502, -0.1387) -> (2.7459, -0.2071) centre (2.913, -0.1833) ccw construction
  arc A80 (2.9918, 0.1534) -> (2.9875, 0.2228) centre (2.8564, 0.1797) ccw construction
  spline S39 degree 4 poles (2.9941, 0.1884) (2.9863, 0.3125) (2.8338, 0.3542) (2.7224, 0.4048) (2.7013, 0.5153) knots 0 0 0 0 0 1 1 1 1 1
  line L129 (2.7095, 0.4723) -> (2.6931, 0.5583) construction
  line L130 (2.9969, 0.1436) -> (2.9913, 0.2332) construction
  arc A81 (2.6983, 0.5497) -> (2.7112, 0.4823) centre (2.867, 0.5469) ccw construction
  arc A82 (2.9918, 0.1534) -> (2.9875, 0.2228) centre (2.8564, 0.1797) ccw construction
  spline S40 degree 4 poles (2.8532, 0.9271) (2.8916, 0.8087) (2.7652, 0.7138) (2.6802, 0.6258) (2.7013, 0.5153) knots 0 0 0 0 0 1 1 1 1 1
  line L131 (2.6931, 0.5583) -> (2.7095, 0.4723) construction
  line L132 (2.8393, 0.9697) -> (2.867, 0.8844) construction
  arc A83 (2.6983, 0.5497) -> (2.7112, 0.4823) centre (2.867, 0.5469) ccw construction
  arc A84 (2.8597, 0.8926) -> (2.8382, 0.9587) centre (2.7219, 0.8844) ccw construction
  spline S41 degree 4 poles (2.8532, 0.9271) (2.8147, 1.0454) (2.6566, 1.0478) (2.5362, 1.0691) (2.4883, 1.1709) knots 0 0 0 0 0 1 1 1 1 1
  line L133 (2.5069, 1.1313) -> (2.4696, 1.2105) construction
  line L134 (2.867, 0.8844) -> (2.8393, 0.9697) construction
  arc A85 (2.4769, 1.2034) -> (2.5061, 1.1414) centre (2.641, 1.2427) ccw construction
  arc A86 (2.8597, 0.8926) -> (2.8382, 0.9587) centre (2.7219, 0.8844) ccw construction
  spline S42 degree 4 poles (2.533, 1.6075) (2.5997, 1.5024) (2.5008, 1.3791) (2.4404, 1.2727) (2.4883, 1.1709) knots 0 0 0 0 0 1 1 1 1 1
  line L135 (2.4696, 1.2105) -> (2.5069, 1.1313) construction
  line L136 (2.5089, 1.6454) -> (2.557, 1.5696) construction
  arc A87 (2.4769, 1.2034) -> (2.5061, 1.1414) centre (2.641, 1.2427) ccw construction
  arc A88 (2.5478, 1.5758) -> (2.5106, 1.6344) centre (2.4165, 1.5335) ccw construction
  spline S43 degree 4 poles (2.533, 1.6075) (2.4663, 1.7125) (2.3126, 1.6756) (2.1906, 1.6663) (2.1189, 1.7529) knots 0 0 0 0 0 1 1 1 1 1
  line L137 (2.1468, 1.7192) -> (2.091, 1.7867) construction
  line L138 (2.557, 1.5696) -> (2.5089, 1.6454) construction
  arc A89 (2.0998, 1.7816) -> (2.1435, 1.7287) centre (2.2489, 1.8605) ccw construction
  arc A90 (2.5478, 1.5758) -> (2.5106, 1.6344) centre (2.4165, 1.5335) ccw construction
  spline S44 degree 4 poles (2.0536, 2.1869) (2.1443, 2.1017) (2.0792, 1.9576) (2.0472, 1.8396) (2.1189, 1.7529) knots 0 0 0 0 0 1 1 1 1 1
  line L139 (2.091, 1.7867) -> (2.1468, 1.7192) construction
  line L140 (2.0209, 2.2176) -> (2.0864, 2.1562) construction
  arc A91 (2.0998, 1.7816) -> (2.1435, 1.7287) centre (2.2489, 1.8605) ccw construction
  arc A92 (2.0759, 2.1599) -> (2.0253, 2.2075) centre (1.9592, 2.0863) ccw construction
  spline S45 degree 4 poles (2.0536, 2.1869) (1.9629, 2.2721) (1.8232, 2.1981) (1.7074, 2.1587) (1.6164, 2.2248) knots 0 0 0 0 0 1 1 1 1 1
  line L141 (1.6518, 2.1991) -> (1.581, 2.2505) construction
  line L142 (2.0864, 2.1562) -> (2.0209, 2.2176) construction
  arc A93 (1.5907, 2.2478) -> (1.6462, 2.2075) centre (1.7156, 2.3613) ccw construction
  arc A94 (2.0759, 2.1599) -> (2.0253, 2.2075) centre (1.9592, 2.0863) ccw construction
  spline S46 degree 4 poles (1.4453, 2.6289) (1.5543, 2.569) (1.5271, 2.4132) (1.5254, 2.2909) (1.6164, 2.2248) knots 0 0 0 0 0 1 1 1 1 1
  line L143 (1.581, 2.2505) -> (1.6518, 2.1991) construction
  line L144 (1.4059, 2.6505) -> (1.4846, 2.6073) construction
  arc A95 (1.5907, 2.2478) -> (1.6462, 2.2075) centre (1.7156, 2.3613) ccw construction
  arc A96 (1.4736, 2.6083) -> (1.4127, 2.6418) centre (1.3788, 2.508) ccw construction
  spline S47 degree 4 poles (1.4453, 2.6289) (1.3362, 2.6889) (1.2193, 2.5824) (1.1169, 2.5155) (1.0123, 2.5569) knots 0 0 0 0 0 1 1 1 1 1
  line L145 (1.0531, 2.5408) -> (0.9716, 2.573) construction
  line L146 (1.4846, 2.6073) -> (1.4059, 2.6505) construction
  arc A97 (0.9817, 2.5728) -> (1.0455, 2.5475) centre (1.0745, 2.7138) ccw construction
  arc A98 (1.4736, 2.6083) -> (1.4127, 2.6418) centre (1.3788, 2.508) ccw construction
  spline S48 degree 4 poles (0.7461, 2.9057) (0.8666, 2.8748) (0.879, 2.7172) (0.9078, 2.5983) (1.0123, 2.5569) knots 0 0 0 0 0 1 1 1 1 1
  line L147 (0.9716, 2.573) -> (1.0531, 2.5408) construction
  line L148 (0.7026, 2.9169) -> (0.7895, 2.8946) construction
  arc A99 (0.9817, 2.5728) -> (1.0455, 2.5475) centre (1.0745, 2.7138) ccw construction
  arc A100 (0.7786, 2.8928) -> (0.7113, 2.9101) centre (0.7118, 2.7721) ccw construction
  spline S49 degree 4 poles (0.7461, 2.9057) (0.6256, 2.9367) (0.5388, 2.8045) (0.4562, 2.7142) (0.3447, 2.7283) knots 0 0 0 0 0 1 1 1 1 1
  line L149 (0.3881, 2.7228) -> (0.3012, 2.7338) construction
  line L150 (0.7895, 2.8946) -> (0.7026, 2.9169) construction
  arc A101 (0.3111, 2.7361) -> (0.3791, 2.7275) centre (0.3658, 2.8957) ccw construction
  arc A102 (0.7786, 2.8928) -> (0.7113, 2.9101) centre (0.7118, 2.7721) ccw construction
  circle A103 centre (0, 0) radius 3.05
  point P0 (-10, -10)
  point P1 (10, 0)
  point P2 (0.1798, 2.8583)
  point P3 (-0.1798, 2.8583)
  point P4 (-0.5366, 2.8132)
  point P5 (-0.885, 2.7237)
  point P6 (-1.2194, 2.5913)
  point P7 (-1.5346, 2.4181)
  point P8 (-1.8255, 2.2067)
  point P9 (-2.0877, 1.9605)
  point P10 (-2.3169, 1.6834)
  point P11 (-2.5097, 1.3797)
  point P12 (-2.6628, 1.0543)
  point P13 (-2.7739, 0.7122)
  point P14 (-2.8413, 0.3589)
  point P15 (-2.8639, 0)
  point P16 (-2.8413, -0.3589)
  point P17 (-2.7739, -0.7122)
  point P18 (-2.6628, -1.0543)
  point P19 (-2.5097, -1.3797)
  point P20 (-2.3169, -1.6834)
  point P21 (-2.0877, -1.9605)
  point P22 (-1.8255, -2.2067)
  point P23 (-1.5346, -2.4181)
  point P24 (-1.2194, -2.5913)
  point P25 (-0.885, -2.7237)
  point P26 (-0.5366, -2.8132)
  point P27 (-0.1798, -2.8583)
  point P28 (0.1798, -2.8583)
  point P29 (0.5366, -2.8132)
  point P30 (0.885, -2.7237)
  point P31 (1.2194, -2.5913)
  point P32 (1.5346, -2.4181)
  point P33 (1.8255, -2.2067)
  point P34 (2.0877, -1.9605)
  point P35 (2.3169, -1.6834)
  point P36 (2.5097, -1.3797)
  point P37 (2.6628, -1.0543)
  point P38 (2.7739, -0.7122)
  point P39 (2.8413, -0.3589)
  point P40 (2.8639, 0)
  point P41 (2.8413, 0.3589)
  point P42 (2.7739, 0.7122)
  point P43 (2.6628, 1.0543)
  point P44 (2.5097, 1.3797)
  point P45 (2.3169, 1.6834)
  point P46 (2.0877, 1.9605)
  point P47 (1.8255, 2.2067)
  point P48 (1.5346, 2.4181)
  point P49 (1.2194, 2.5913)
  point P50 (0.885, 2.7237)
  point P51 (0.5366, 2.8132)
  point P52 (-1.0123, 2.5569)
  point P53 (-1.6164, 2.2248)
  point P54 (-2.1189, 1.7529)
  point P55 (-2.4883, 1.1709)
  point P56 (-2.7013, 0.5153)
  point P57 (-2.7446, -0.1727)
  point P58 (-2.6154, -0.8498)
  point P59 (-2.3219, -1.4735)
  point P60 (-1.8825, -2.0047)
  point P61 (-1.3248, -2.4098)
  point P62 (-0.6839, -2.6636)
  point P63 (0, -2.75)
  point P64 (1.3248, -2.4098)
  point P65 (1.8825, -2.0047)
  point P66 (2.3219, -1.4735)
  point P67 (2.6154, -0.8498)
  point P68 (2.7446, -0.1727)
  point P69 (2.7013, 0.5153)
  point P70 (2.4883, 1.1709)
  point P71 (2.1189, 1.7529)
  point P72 (1.6164, 2.2248)
  point P73 (1.0123, 2.5569)
  point P74 (0.3447, 2.7283)
  dimension "d41" = 13
  dimension "d42" = 11
  dimension "d45" = 10
  dimension "d46" = 10
  dimension "d49" = 360
  dimension "d53" = 360
  dimension "d63" = 6.1
  constraints: 300 end point, 103 centre point, 102 midpoint, 101 point on circle, 2 coincident, 1154 other
  measures "d41" diameter of A0
  measures "d42" diameter of A1
  measures "d45" distance of point (10, 0) A0.centre
  measures "d46" distance from line of L0 A0.centre
  measures "d63" diameter of A103
extrude "Extrusion10" cut sketch "Skizze4" against normal blind 4 contours S0 S49 S48 S47 S46 S45 S44 S43 S42 S41 S40 S39 S38 S37 S36 S35 S34 S33 S32 S31 S30 S29 S28 S27 S26 S25 S24 S23 S22 S21 S20 S19 S18 S17 S16 S15 S14 S13 S12 S11 S10 S9 S8 S7 S6 S5 S4 S3 S2 S1 | A103
extrude "Extrusion8" add sketch "Skizze4" along normal blind 1 contours A0
extrude "Extrusion9" add sketch "Skizze4" along normal blind 2 contours A1
chamfer "Fase1" distance 2 angle 45 4 edges at (-18.5, 20, 0) (-18.5, 10, 20) (-18.5, 0, 0) (-18.5, 10, -20)
fillet "Rundung2" radius 1 4 edges at (1, 20, -20) (1, 0, -20) (1, 20, 20) (1, 0, 20)
fillet "Rundung3" radius 2 4 edges at (12.5, 19, -27) (12.5, 1, -27) (12.5, 19, 27) (12.5, 1, 27)
equation "\"PrintTol\" = 0.1"
